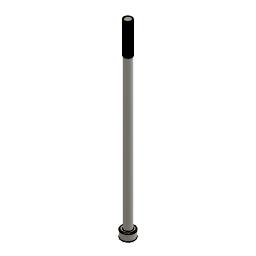
Tige_filetéeM6_14.5 (Autodesk Fusion 360 design; units mm, degrees)
part number: 2026-08-19-09-42-57-255
Autodesk Fusion 360 part; units mm, degrees
sketch "Esquisse1" plane through (0, 0, 0) normal (0, 1, 0) x (1, 0, 0)
  circle A0 centre (0, 0) radius 3
  circle A1 centre (0, 0) radius 5
  dimension "d1" = 6
  dimension "d4" = 10
  constraint coincident A0.centre A1.centre
  constraint concentric A0 A1
  measures "d1" diameter of A0
  measures "d4" diameter of A1
extrude "Extrusion1" add sketch "Esquisse1" along normal blind 115 contours A0 makes body 1
extrude "Extrusion2" add sketch "Esquisse1" against normal blind 6 separate body contours A0 | A1 makes body 2
extrude "Extrusion3" add 1 faces at (-1.1591, 115, -0.5829) along direction (0, 1, 0) blind 24 separate body on bodies 1 makes body 3
thread "Filetage1" "ISO Metric profile 6.0 M6x0.7 M6x0.7 6g" major diameter 5.908 minor diameter 5.1087 pitch 0.7 angle 60 modelled right hand crest width 0.1005 on face at (2.9963, 131, 0.1495) crest through (2.954, 114.825, 0) on bodies 3
sketch "Esquisse2" plane through (0, -6, 0) normal (0, -1, 0) x (1, 0, 0)
  circle A0 centre (0, 0) radius 5
  line L0 (-3.087, 0.7443) -> (-2.1881, -2.3012)
  line L1 (-2.1881, -2.3012) -> (0.8989, -3.0455)
  line L2 (0.8989, -3.0455) -> (3.087, -0.7443)
  line L3 (3.087, -0.7443) -> (2.1881, 2.3012)
  line L4 (2.1881, 2.3012) -> (-0.8989, 3.0455)
  line L5 (-0.8989, 3.0455) -> (-3.087, 0.7443)
  dimension "d11" = 5.5
  constraint coincident A0.centre origin
  measures "d11" distance of L1 L4
extrude "Extrusion4" cut sketch "Esquisse2" against normal blind 4 contours L0 L1 L2 L3 L4 L5 bodies 2
fillet "Congé1" radius 2 6 edges at (0.6446, -2, 2.6734) (-1.9929, -2, 1.8949) (-2.6375, -2, -0.7785) (-0.6446, -2, -2.6734) (1.9929, -2, -1.8949) (2.6375, -2, 0.7785) on bodies 2
fillet "Congé2" radius 0.5 2 edges at (-4.6616, -6, -1.8081) (-4.6616, 0, 1.8081) on bodies 2
